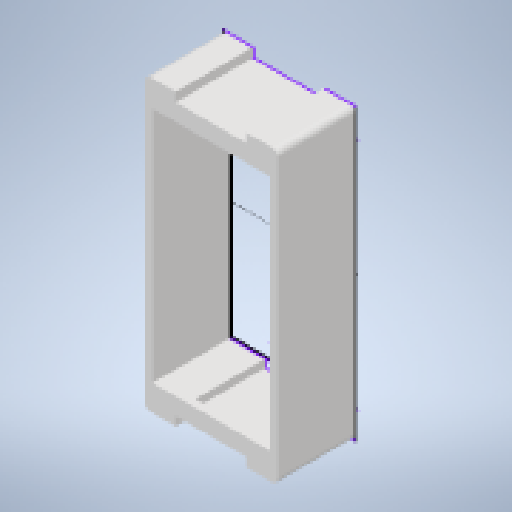
# Autodesk Inventor part: fast_akkum
Saved by Autodesk Inventor 2023 (Build 270158000, 158)
## iProperties
Created: 2026-02-16
Part Number: fast_akkum
Material: Типовые
Document SubType Name: Modeling
Designer: garin
Density: 1 g/cm^3
Appearance: По умолчанию
Author: garin
Autodesk Inventor part; units mm, degrees
ref_plane "YZ Plane" through (0, 0, 0) normal (1, 0, 0) x (0, 1, 0)
ref_plane "XZ Plane" through (0, 0, 0) normal (0, 1, 0) x (-1, 0, 0)
ref_plane "XY Plane" through (0, 0, 0) normal (0, 0, 1) x (1, 0, 0)
sketch "Эскиз1" plane through (0, 0, 0) normal (0, 0, 1) x (1, 0, 0)
  line L0 (-18.25, -37.6) -> (18.25, -37.6)
  line L1 (18.25, -37.6) -> (18.25, 37.6)
  line L2 (18.25, 37.6) -> (-18.25, 37.6)
  line L3 (-18.25, 37.6) -> (-18.25, -37.6)
  line L4 (-18.25, 0) -> (18.25, 0) construction
  line L5 (0, 37.6) -> (0, -37.6) construction
  line L6 (-18.45, -37.8) -> (18.45, -37.8)
  line L7 (18.45, -37.8) -> (18.45, 37.8)
  line L8 (18.45, 37.8) -> (-18.45, 37.8)
  line L9 (-18.45, 37.8) -> (-18.45, -37.8)
  line L10 (-7.5, -37.8) -> (7.5, -37.8)
  line L11 (7.5, -37.8) -> (7.5, -40.8)
  line L12 (7.5, -40.8) -> (-7.5, -40.8)
  line L13 (-7.5, -40.8) -> (-7.5, -37.8)
  line L14 (-18.45, -37.8) -> (-18.45, -43.8)
  line L15 (-18.45, -43.8) -> (18.45, -43.8)
  line L16 (18.45, -43.8) -> (18.45, -37.8)
  line L17 (-18.45, 37.8) -> (-18.45, 43.8)
  line L18 (-18.45, 43.8) -> (18.45, 43.8)
  line L19 (18.45, 43.8) -> (18.45, 37.8)
  line L20 (-18.45, -43.8) -> (-21.45, -43.8)
  line L21 (-21.45, -43.8) -> (-21.45, 43.8)
  line L22 (-21.45, 43.8) -> (-18.45, 43.8)
  line L23 (-18.45, 43.8) -> (-18.45, -43.8)
  line L24 (18.45, 37.8) -> (18.45, 43.8)
  line L25 (21.45, -43.8) -> (21.45, 43.8)
  line L26 (21.45, 43.8) -> (18.45, 43.8)
  line L27 (18.45, 43.8) -> (18.45, -43.8)
  line L28 (7.5, 37.8) -> (7.5, 40.8)
  line L29 (7.5, 40.8) -> (-7.5, 40.8)
  line L30 (-7.5, 40.8) -> (-7.5, 37.8)
  line L31 (-21.45, -43.8) -> (-11.45, -43.8)
  line L32 (18.45, -43.8) -> (21.45, -43.8)
  line L33 (21.45, -43.8) -> (11.45, -43.8)
  line L34 (16.45, 46.7) -> (21.45, 46.7)
  line L35 (16.45, 46.7) -> (11.45, 46.7)
  line L36 (11.45, 46.7) -> (11.45, 43.8)
  line L37 (21.45, 46.7) -> (21.45, 43.8)
  line L38 (11.45, 43.8) -> (16.45, 43.8)
  circle A0 centre (16.45, 43.8) radius 2.1
  line L39 (-16.45, 46.7) -> (-21.45, 46.7)
  line L40 (-16.45, 46.7) -> (-11.45, 46.7)
  line L41 (-11.45, 46.7) -> (-11.45, 43.8)
  line L42 (-21.45, 46.7) -> (-21.45, 43.8)
  circle A1 centre (-16.45, 43.8) radius 2.1
  line L43 (16.45, -46.7) -> (21.45, -46.7)
  line L44 (16.45, -46.7) -> (11.45, -46.7)
  line L45 (11.45, -46.7) -> (11.45, -43.8)
  line L46 (21.45, -46.7) -> (21.45, -43.8)
  circle A2 centre (16.45, -43.8) radius 2.1
  line L47 (-11.45, -46.7) -> (-11.45, -43.8)
  line L48 (-16.45, -46.7) -> (-11.45, -46.7)
  line L49 (-16.45, -46.7) -> (-21.45, -46.7)
  line L50 (-21.45, -46.7) -> (-21.45, -43.8)
  circle A3 centre (-16.45, -43.8) radius 2.1
  line L51 (-18.45, -37.8) -> (-18.95, -37.8)
  line L52 (-18.95, -37.8) -> (-18.95, -38.3)
  line L53 (-18.95, -38.3) -> (-18.45, -38.3)
  line L54 (-18.45, -38.3) -> (-18.45, -37.8)
  line L55 (-18.95, -38.3) -> (18.95, -38.3)
  line L56 (18.95, -38.3) -> (18.95, 38.3)
  line L57 (18.95, 38.3) -> (-18.95, 38.3)
  line L58 (-18.95, 38.3) -> (-18.95, -38.3)
  point P0 (0, 0)
  point P1 (0, 0)
  point P2 (-1.9914, -32.8601)
  point P3 (0, -37.8)
  dimension "d0" = 36.5
  dimension "d1" = 75.2
  dimension "d4" = 36.9
  dimension "d5" = 75.6
  dimension "d6" = 15
  dimension "d7" = 3
  dimension "d9" = 6
  dimension "d10" = 3
  dimension "d18" = 5
  dimension "d19" = 4.2
  dimension "d27" = 0.5
  dimension "d28" = 0.5
  dimension "d29" = 37.9
  dimension "d30" = 76.6
  constraints: 118 end point, 23 symmetric about line, 12 parallel, 10 perpendicular, 8 horizontal, 6 midpoint, 6 point on line, 4 centre point, 2 coincident, 2 vertical, 3 other
  measures "d0" distance of L2.end L1.end
  measures "d1" distance of L1.end L0.end
  measures "d4" distance of L8.end L7.end
  measures "d5" distance of L7.end L6.end
  measures "d6" distance of L11.end L12.end
  measures "d7" distance of L10.end L11.end
  measures "d9" distance of L6.start L14.end
  measures "d10" distance of L21.end L22.end
  measures "d18" distance of L36.end L38.end
  measures "d19" diameter of A0
  measures "d27" distance of L53.end L52.end
  measures "d28" distance of L52.end L51.end
  measures "d29" distance of L57.end L56.end
  measures "d30" distance of L56.end L55.end
extrude "Выдавливание1" add sketch "Эскиз1" along normal blind 25 contours L55 L13 L12 L11 L16 A2 L15 A3 L14 | L14 A3 L20 L21 L22 A1 L17 L57 L58 L52 L53 | L55 L11 L12 L13 | L17 A1 L18 A0 L19 L57 L28 L29 L30 | A3 L15 L14 | L14 L20 A3 | L30 L29 L28 L57 | A1 L22 L17 | L17 L18 A1 | L15 A3 L20 | L15 L47 L48 L49 L50 L20 A3 | L55 L56 L57 L19 A0 L26 L25 L32 A2 L16 | L22 A1 L18 | L22 L42 L39 L40 L41 L18 A1 | A2 L32 L16 | L16 L15 A2 | L15 A2 L32 L46 L43 L44 L45 | A0 L18 L19 | L19 L26 A0 | L32 A2 L15 | L36 L35 L34 L37 L26 A0 L18 | L18 A0 L26
extrude "Выдавливание2" cut sketch "Эскиз1" along normal blind 8 contours A3 L15 L14 | L14 L20 A3 | A1 L22 L17 | L17 L18 A1 | L15 A3 L20 | L22 A1 L18 | A2 L32 L16 | L16 L15 A2 | A0 L18 L19 | L19 L26 A0 | L32 A2 L15 | L18 A0 L26
extrude "Выдавливание3" cut sketch "Эскиз1" along normal blind 22.5 contours L6 L11 L55 L13 | L55 L11 L12 L13 | L30 L57 L28 L8 | L30 L29 L28 L57
fillet "Сопряжение1" radius 2 4 edges at (21.45, -46.7, 12.5) (-21.45, -46.7, 12.5) (-21.45, 46.7, 12.5) (21.45, 46.7, 12.5)
